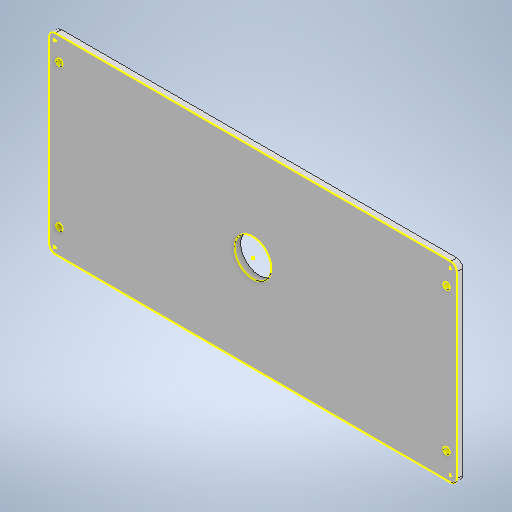
# Autodesk Inventor part: canon_plate
Saved by Autodesk Inventor 2025.1 (Build 291241000, 241)
## iProperties
Created: 2024-10-05
Part Number: canon_plate
Material: 一般
Document SubType Name: Modeling
Designer: yuki0520
Density: 1 g/cm^3
Appearance: 既定
Author: yuki0520
Autodesk Inventor part; units mm, degrees
ref_plane "YZ Plane" through (0, 0, 0) normal (1, 0, 0) x (0, 1, 0)
ref_plane "XZ Plane" through (0, 0, 0) normal (0, 1, 0) x (-1, 0, 0)
ref_plane "XY Plane" through (0, 0, 0) normal (0, 0, 1) x (1, 0, 0)
sketch "スケッチ1" plane through (0, 0, 0) normal (0, 0, 1) x (1, 0, 0)
  circle A0 centre (0, 0) radius 9
  circle A1 centre (0, 0) radius 77
  line L0 (100, -77) -> (-100, -77)
  line L1 (-100, -77) -> (-100, 77)
  line L2 (-100, 77) -> (100, 77)
  line L3 (100, 77) -> (100, -77)
  line L4 (100, -77) -> (-100, 77) construction
  line L5 (-100, -77) -> (100, 77) construction
  line L6 (-100, 47) -> (100, 47)
  circle A2 centre (-95, -34.5) radius 1.6
  circle A3 centre (-95, 35.5) radius 1.6
  circle A4 centre (95, 35.5) radius 1.6
  circle A5 centre (95, -34.5) radius 1.6
  line L7 (-100, -47) -> (100, -47)
  dimension "d0" = 18
  dimension "d1" = 154
  dimension "d2" = 200
  dimension "d3" = 30
  dimension "d4" = 3.2
  dimension "d5" = 3.2
  dimension "d6" = 3.2
  dimension "d7" = 3.2
  dimension "d9" = 5
  dimension "d11" = 5
  dimension "d12" = 70
  dimension "d13" = 5
  dimension "d15" = 5
  dimension "d16" = 70
  dimension "d19" = 11.5
  dimension "d20" = 11.5
  dimension "d21" = 30
  constraints: 16 end point, 6 centre point, 4 point on line, 3 perpendicular, 2 coincident, 2 midpoint, 2 parallel, 1 horizontal, 1 tangent
  measures "d0" diameter of A0
  measures "d1" diameter of A1
  measures "d2" distance of L1.end L2.end
  measures "d3" distance between parallel lines of L2 L6
  measures "d4" diameter of A2
  measures "d5" diameter of A3
  measures "d6" diameter of A4
  measures "d7" diameter of A5
  measures "d9" distance from line of L1 A2.centre
  measures "d11" distance from line of L1 A3.centre
  measures "d12" distance of A2.centre A3.centre
  measures "d13" distance from line of L3 A5.centre
  measures "d15" distance from line of L3 A4.centre
  measures "d16" distance of A5.centre A4.centre
  measures "d19" distance from line of L6 A3.centre
  measures "d20" distance from line of L6 A4.centre
  measures "d21" distance between parallel lines of L0 L7
extrude "押し出し1" add sketch "スケッチ1" along normal blind 3 contours A1 L7 L6 | A1 L6 L3 L7 | A1 L7 L1 L6
fillet "フィレット1" radius 3 4 edges at (100, 47, 1.5) (100, -47, 1.5) (-100, -47, 1.5) (-100, 47, 1.5)
sketch "スケッチ2" plane through (0, 0, 3) normal (0, 0, 1) x (1, 0, 0)
  arc A0 (-97, 47) -> (-100, 44) centre (-97, 44) ccw projected
  line L0 (-100, 44) -> (-100, -44) projected
  arc A1 (-100, -44) -> (-97, -47) centre (-97, -44) ccw projected
  line L1 (-97, -47) -> (97, -47) projected
  arc A2 (97, -47) -> (100, -44) centre (97, -44) ccw projected
  line L2 (100, -44) -> (100, 44) projected
  arc A3 (100, 44) -> (97, 47) centre (97, 44) ccw projected
  line L3 (97, 47) -> (-97, 47) projected
  circle A4 centre (-95, -34.5) radius 1.6 projected
  circle A5 centre (-95, 35.5) radius 1.6 projected
  circle A6 centre (0, 0) radius 9 projected
  circle A7 centre (95, -34.5) radius 1.6 projected
  circle A8 centre (95, 35.5) radius 1.6 projected
equation "\"d16\" = d12"
equation "\"d20\" = d19"
equation "\"d21\" = d3"
